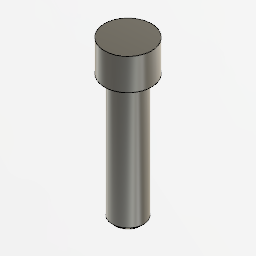
Cap_Screw (Autodesk Fusion 360 design; units mm, degrees)
Autodesk Fusion 360 part; units mm, degrees
sketch "Sketch1" plane through (0, 0, 0) normal (0, 1, 0) x (1, 0, 0)
  line L0 (0, 0) -> (0, -12.7)
  line L1 (0, -12.7) -> (9.525, -12.7)
  line L2 (9.525, -12.7) -> (9.525, 0)
  line L3 (9.525, 0) -> (6.35, 0)
  line L4 (6.35, 0) -> (6.35, 49.53)
  line L5 (6.35, 49.53) -> (5.08, 50.8)
  line L6 (5.08, 50.8) -> (0, 50.8)
  line L7 (0, 50.8) -> (0, 0)
  dimension "headradius" = 9.525
  dimension "radius" = 6.35
  dimension "headheight" = 12.7
  dimension "length" = 50.8
  dimension "chamferangle" = 45
  dimension "chamfersize" = 1.27
  measures "headradius" distance of L0 L2
  measures "radius" distance of L4 L7
  measures "headheight" distance of L1 L3
  measures "length" distance of L0.start L6
  measures "chamferangle" angle of L5 L6
  measures "chamfersize" distance of L4.end L6
revolve "Revolve1" add sketch "Sketch1" angle 360 about axis through (0, 0, 0) along (0, 0, 1)
equation "chamfersize = radius / 5"
